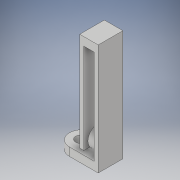
# Autodesk Inventor part: Smaller ethernet holder
Saved by Autodesk Inventor 2018 (Build 220112000, 112)
## iProperties
Created: 2019-10-02
Part Number: Smaller ethernet holder
Material: Generic
Document SubType Name: Modeling
Designer: Jacob
Density: 1 g/cm^3
Appearance: Default
Author: Jacob
Autodesk Inventor part; units mm, degrees
ref_plane "YZ Plane" through (0, 0, 0) normal (1, 0, 0) x (0, 1, 0)
ref_plane "XZ Plane" through (0, 0, 0) normal (0, 1, 0) x (-1, 0, 0)
ref_plane "XY Plane" through (0, 0, 0) normal (0, 0, 1) x (1, 0, 0)
sketch "Sketch1" plane through (0, 0, 0) normal (0, 1, 0) x (-1, 0, 0)
  line L0 (2.25, 3) -> (-2.25, 3)
  line L1 (-2.25, 3) -> (-2.25, -3)
  line L2 (-2.25, -3) -> (2.25, -3)
  line L3 (2.25, -3) -> (2.25, 3)
  line L4 (2.25, 3) -> (-2.25, -3) construction
  line L5 (-2.25, 3) -> (2.25, -3) construction
  point P0 (0, 0)
  dimension "d0" = 6
  dimension "d1" = 4.5
  constraints: 12 end point, 2 midpoint, 2 parallel, 1 horizontal, 1 perpendicular
  measures "d0" distance of L2.end L0.start
  measures "d1" distance of L1.end L2.end
extrude "Extrusion1" add sketch "Sketch1" along normal blind 2
sketch "Sketch2" plane through (0, 0, 0) normal (0, -1, 0) x (1, 0, 0)
  line L0 (-2.25, -3) -> (-2.25, 3) projected
  line L1 (-2.25, 0) -> (2.25, 0) construction
  line L2 (2.25, 3) -> (2.25, -3) projected
  line L3 (0, 3) -> (0, -3) construction
  line L4 (2.25, -3) -> (-2.25, -3) projected
  line L5 (-2.25, 3) -> (2.25, 3) projected
  line L6 (-2.25, 3) -> (-1.25, 3)
  line L7 (-1.25, 3) -> (-1.25, -3)
  line L8 (-1.25, -3) -> (-2.25, -3)
  line L9 (-2.25, -3) -> (-2.25, 3)
  line L10 (2.25, 3) -> (1.25, 3)
  line L11 (1.25, 3) -> (1.25, -3)
  line L12 (1.25, -3) -> (2.25, -3)
  line L13 (2.25, -3) -> (2.25, 3)
  point P0 (0, 0)
  dimension "d4" = 1
  dimension "d5" = 1
  constraints: 20 end point, 4 parallel, 3 midpoint, 2 horizontal, 2 perpendicular, 2 point on line
  measures "d4" distance between parallel lines of L0 L7
  measures "d5" distance between parallel lines of L2 L11
extrude "Extrusion2" add sketch "Sketch2" along normal blind 22 contours L0 L5 L7 L4 | L11 L5 L2 L4
sketch "Sketch3" plane through (0, -22, 0) normal (0, -1, 0) x (1, 0, 0)
  line L0 (-1.25, 3) -> (1.25, 3) projected
  line L1 (2.25, 3) -> (2.25, -3) projected
  line L2 (1.25, 3) -> (2.25, 3)
  line L3 (2.25, 3) -> (2.25, -3)
  line L4 (2.25, -3) -> (1.25, -3)
  line L5 (1.25, -3) -> (1.25, 3)
  point P0 (0, 0)
  constraints: 8 end point, 2 parallel, 1 horizontal, 1 perpendicular
extrude "Extrusion3" add sketch "Sketch3" along normal blind 3
sketch "Sketch4" plane through (1.25, 0, -3) normal (-1, 0, 0) x (0, 0, 1)
  line L0 (0, -25) -> (6, -25) projected
  line L1 (6, 0) -> (6, -25) projected
  line L2 (0, -25) -> (6, -25)
  line L3 (6, -25) -> (6, -23)
  line L4 (6, -23) -> (0, -23)
  line L5 (0, -23) -> (0, -25)
  point P0 (3, 0)
  dimension "d10" = 2
  constraints: 8 end point, 2 parallel, 1 horizontal, 1 perpendicular, 1 point on line
  measures "d10" distance between parallel lines of L0 L4
extrude "Extrusion4" add sketch "Sketch4" along normal blind 9
sketch "Sketch5" plane through (1.25, -23, 3) normal (0, 1, 0) x (1, 0, 0)
  line L0 (-9, 0) -> (-9, 6) projected
  line L1 (-9, 3) -> (-3.5, 3) construction
  line L2 (-3.5, 6) -> (-3.5, 0) projected
  line L3 (0, 6) -> (-9, 6) projected
  line L4 (-6.25, 6) -> (-6.25, 3) construction
  line L5 (-6.25, 3) -> (-6.25, 0) construction
  line L6 (1, 0) -> (-9, 0) projected
  circle A0 centre (-6.25, 3) radius 1.25
  point P0 (-1.25, 3)
  dimension "d13" = 2.5
  constraints: 6 end point, 3 midpoint, 2 point on line, 1 centre point, 1 coincident, 1 vertical
  measures "d13" diameter of A0
extrude "Extrusion5" cut sketch "Sketch5" against normal blind 3.5 contours A0
sketch "Sketch6" plane through (1.25, 0, -3) normal (-1, 0, 0) x (0, 0, 1)
  line L0 (6, 0) -> (6, -23) projected
  line L1 (6, -17.5) -> (0, -17.5)
  line L2 (0, -25) -> (0, 2) projected
  line L3 (0, 0) -> (6, 0) projected
  line L4 (6, -20) -> (0, -20)
  line L5 (0, 0) -> (0, -23) projected
  circle A0 centre (3, -20) radius 2.5
  circle A1 centre (3, -20) radius 1
  point P0 (3, 0)
  dimension "d16" = 17.5
  dimension "d17" = 2.5
  dimension "d18" = 5
  dimension "d19" = 2
  constraints: 4 end point, 4 point on line, 2 centre point, 1 coincident, 1 horizontal, 1 midpoint, 1 perpendicular
  measures "d16" distance between parallel lines of L3 L1
  measures "d17" distance between parallel lines of L1 L4
  measures "d18" diameter of A0
  measures "d19" diameter of A1
extrude "Extrusion6" add sketch "Sketch6" along normal blind 2 contours A0 L4 A1 | A0 L4 A1
sketch "Sketch7" plane through (-2.25, 2, -3) normal (-1, 0, 0) x (0, 0, 1)
  line L0 (0.0186, -19.5) -> (6, -19.5) construction
  line L1 (6, -2) -> (6, -25) projected
  line L2 (0, 0) -> (6, 0) projected
  line L3 (0, -2) -> (0, -24) projected
  line L4 (0, -22) -> (6, -22) construction
  circle A0 centre (3, -22) radius 1
  line L5 (0, -2) -> (6, -2) construction
  line L6 (0, -2) -> (6, -2)
  point P0 (3, -2)
  dimension "d23" = 2.5
  dimension "d24" = 2
  dimension "d25" = 17.5
  constraints: 6 end point, 3 point on line, 1 centre point, 1 collinear, 1 horizontal, 1 midpoint, 1 perpendicular
  measures "d23" distance between parallel lines of L0 L4
  measures "d24" diameter of A0
  measures "d25" distance between parallel lines of L0 L5
extrude "Extrusion7" cut sketch "Sketch7" against normal blind 2
fillet "Fillet1" radius 3 2 edges at (-7.75, -24, 3) (-7.75, -24, -3)
body "Solid1"
